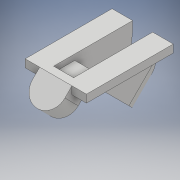
# Autodesk Inventor part: shaft_jig
Saved by Autodesk Inventor 2017 SP1 (Build 210196100, 196)
## iProperties
Part Number: shaft_jig
Material: 一般
Document SubType Name: Modeling
Designer: gisen
Density: 1 g/cm^3
Appearance: 既定
Author: gisen
Autodesk Inventor part; units mm, degrees
ref_plane "YZ Plane" through (0, 0, 0) normal (1, 0, 0) x (0, 1, 0)
ref_plane "XZ Plane" through (0, 0, 0) normal (0, 1, 0) x (-1, 0, 0)
ref_plane "XY Plane" through (0, 0, 0) normal (0, 0, 1) x (1, 0, 0)
sketch "スケッチ1" plane through (0, 0, 0) normal (0, 0, 1) x (1, 0, 0)
  line L0 (-27.5, -39) -> (27.5, -39)
  line L1 (27.5, -39) -> (27.5, 39)
  line L2 (27.5, 39) -> (-27.5, 39)
  line L3 (-27.5, 39) -> (-27.5, -39)
  line L4 (-27.5, -39) -> (27.5, 39) construction
  line L5 (27.5, -39) -> (-27.5, 39) construction
  point P0 (0, 0)
  dimension "d0" = 55
  dimension "d1" = 78
  constraints: 12 end point, 2 midpoint, 2 parallel, 1 horizontal, 1 perpendicular
  measures "d0" distance of L2.end L1.end
  measures "d1" distance of L1.end L0.end
extrude "押し出し1" add sketch "スケッチ1" along normal blind 7
sketch "スケッチ2" plane through (0, 0, 7) normal (0, 0, 1) x (1, 0, 0)
  line L0 (9, -27) -> (9, 39)
  line L1 (9, 39) -> (-9, 39)
  line L2 (-9, 39) -> (-9, -27)
  line L3 (-9, -27) -> (9, -27)
  line L4 (9, -27) -> (-9, 39) construction
  line L5 (9, 39) -> (-9, -27) construction
  point P0 (0, 0)
  point P1 (0, 6)
  dimension "d4" = 18
  dimension "d5" = 66
  dimension "d15" = 9
  constraints: 12 end point, 2 midpoint, 2 parallel, 1 perpendicular
  measures "d4" distance of L1.end L0.end
  measures "d5" distance of L0.start L0.end
  measures "d15" distance from line of L0 point (0, 0)
extrude "押し出し2" cut sketch "スケッチ2" against normal blind 7
ref_plane "作業平面1" through (-27.5, -39, 7) normal (0, 0.7071068, -0.7071068) x (1, 0, 0)
sketch "スケッチ5" plane through (-27.5, -39, 7) normal (0, 0.7071068, -0.7071068) x (1, 0, 0)
  line L0 (0, 4.9497) -> (55, 4.9497) projected
  line L1 (55, 4.9497) -> (55, 0) projected
  line L2 (0, 0) -> (55, 0) projected
  line L3 (0, 4.9497) -> (0, 0) projected
  line L4 (27.5, 9) -> (42, 9) construction
  line L5 (27.5, 9) -> (42, 9) construction
  line L6 (27.5, 9) -> (13, 9) construction
  line L7 (42, 0) -> (13, 0)
  line L8 (13, 0) -> (13, 9)
  line L9 (42, 9) -> (42, 0)
  line L10 (42, 9) -> (13, 9)
  line L11 (13, 9) -> (13, 0)
  line L12 (13, 0) -> (42, 0)
  line L13 (42, 0) -> (42, 9)
  arc A0 (42, 9) -> (13, 9) centre (27.5, 9) ccw
  point P0 (27.5, -22.6274)
  dimension "d14" = 180
  dimension "d16" = 9
  dimension "d17" = 0
  dimension "d18" = 9
  dimension "d19" = 55
  dimension "d20" = 27.5
  constraints: 20 end point, 2 horizontal, 2 parallel, 2 perpendicular, 2 point on circle, 1 centre point, 1 coincident, 1 collinear, 1 vertical
  measures "d14" angle of L6 L4
  measures "d16" distance of L5.end L7.start
  measures "d17" distance between parallel lines of L7 L2
  measures "d18" distance of L7.end L6.end
  measures "d19" distance of L0.start L0.end
  measures "d20" distance from line of L3 L4.start
extrude "押し出し4" add sketch "スケッチ5" along normal blind 17 contours L8 L10 L9 L0 | L0 L9 L2 L8 | A0 L10
sketch "スケッチ6" plane through (-14.5, -26.9792, -5.0208) normal (0, 0.7071068, 0.7071068) x (1, 0, 0)
  line L0 (5.5, -7.1005) -> (23.5, -7.1005) projected
  line L1 (29, -7.1005) -> (0, -7.1005) projected
  line L2 (29, -7.1005) -> (29, 0) projected
  line L3 (0, 0) -> (29, 0) projected
  line L4 (0, -7.1005) -> (0, 0) projected
  line L5 (0, -17) -> (0, 0) projected
  line L6 (29, -7.1005) -> (0, -7.1005)
  line L7 (0, -7.1005) -> (0, 0)
  line L8 (0, 0) -> (29, 0)
  line L9 (29, 0) -> (29, -7.1005)
  point P0 (14.5, 15.5269)
  constraints: 8 end point, 2 parallel, 1 horizontal, 1 perpendicular
extrude "押し出し5" add sketch "スケッチ6" along normal up to surface surface through (0, 0, 0) normal (0, 0, 1)
chamfer "面取り1" distance 5 angle 45 1 edges at (0, -27, 7)
sketch "スケッチ8" plane through (-9, -21.9584, 0) normal (0, 0, 1) x (1, 0, 0)
  line L0 (18, -5.0416) -> (18, 0) projected
  line L1 (0, 0) -> (18, 0) projected
  line L2 (0, 0) -> (0, -5.0416) projected
  line L3 (0, -5.0416) -> (18, -5.0416) projected
  line L4 (0, -5.0416) -> (18, -5.0416) projected
  line L5 (0, -5.0416) -> (18, -5.0416)
  line L6 (18, -5.0416) -> (18, 8.9584)
  line L7 (18, 8.9584) -> (0, 8.9584)
  line L8 (0, 8.9584) -> (0, -5.0416)
  point P0 (9, 21.9584)
  dimension "d30" = 14
  constraints: 8 end point, 2 parallel, 1 horizontal, 1 perpendicular
  measures "d30" distance of L6.end L5.end
extrude "押し出し8" add sketch "スケッチ8" along normal blind 2
ref_plane "作業平面2" through (-27.5, 1.3051, -33.3051) normal (0, 0.7071068, -0.7071068) x (-1, 0, 0)
ref_plane "作業平面3" through (7.25, -21.9584, 0) normal (0, 0.7071068, 0.7071068) x (1, 0, 0)
sketch "スケッチ9" plane through (7.25, -21.9584, 0) normal (0, 0.7071068, 0.7071068) x (1, 0, 0)
  line L0 (-21.75, 0) -> (-21.75, -12.0503) projected
  line L1 (-34.75, -12.0503) -> (-21.75, -12.0503) projected
  line L2 (-34.75, 43.1041) -> (-34.75, -12.0503) projected
  line L3 (-16.25, 43.1041) -> (-34.75, 43.1041) projected
  line L4 (-16.25, 43.1041) -> (-16.25, 6.3345) projected
  line L5 (1.75, 6.3345) -> (-16.25, 6.3345) construction
  line L6 (1.75, 6.3345) -> (1.75, 43.1041) projected
  line L7 (20.25, 43.1041) -> (1.75, 43.1041) projected
  line L8 (20.25, -12.0503) -> (20.25, 43.1041) projected
  line L9 (7.25, -12.0503) -> (20.25, -12.0503) projected
  line L10 (7.25, -12.0503) -> (7.25, 0) projected
  line L11 (-21.75, 0) -> (7.25, 0) projected
  line L12 (-7.25, 50) -> (6, 50) construction
  line L13 (-7.25, 50) -> (6, 50) construction
  line L14 (-7.25, 50) -> (-20.5, 50) construction
  line L15 (7.25, 0) -> (-21.75, 0) projected
  line L16 (6, 50) -> (6, 0)
  line L17 (-20.5, 50) -> (-20.5, 0)
  line L18 (6, 0) -> (-20.5, 0)
  line L19 (-20.5, 0) -> (6, 0)
  arc A0 (6, 50) -> (-20.5, 50) centre (-7.25, 50) ccw
  point P0 (-7.25, 15.5269)
  dimension "d40" = 50
  dimension "d41" = 26.5
  constraints: 14 end point, 3 perpendicular, 2 collinear, 2 point on circle, 2 point on line, 1 centre point, 1 coincident, 1 horizontal
  measures "d40" distance of L13.end L16.end
  measures "d41" distance between parallel lines of L17 L16
extrude "押し出し9" add sketch "スケッチ9" along normal up to surface contours L17 A0 L16 L11 surface through (0, 0, 0) normal (0, 0, 1)
sketch "スケッチ10" plane through (13.25, -21.9584, 0) normal (1, 0, 0) x (0, 0, -1)
  line L0 (-7, -17.0416) -> (0, -17.0416) projected
  line L1 (-7, -17.0416) -> (-0.636, -23.4056) projected
  line L2 (-0.636, -23.4056) -> (11.3848, -11.3848) projected
  line L3 (11.3848, -11.3848) -> (0, 0) projected
  line L4 (0, -17.0416) -> (0, 0) projected
  line L5 (0, 70.7107) -> (0, 60.9584) projected
  line L6 (0, 0) -> (0, 60.9584) projected
  line L7 (0, 0) -> (35.3553, 35.3553) projected
  line L8 (35.3553, 35.3553) -> (0, 70.7107) projected
  line L9 (0, -7.8048) -> (7, -7.8048)
  line L10 (7, -7.8048) -> (7, 11.1857)
  line L11 (7, 11.1857) -> (0, 11.1857)
  line L12 (0, 11.1857) -> (0, -7.8048)
  line L13 (0, -17.0416) -> (0, 60.9584) projected
  line L14 (0, 60.9584) -> (-7, 60.9584) projected
  line L15 (-7, -17.0416) -> (-7, 60.9584) projected
  line L16 (0, -17.0416) -> (-7, -17.0416) projected
  line L17 (0, -17.0416) -> (0, 60.9584) projected
  point P0 (0, 21.9584)
  dimension "d44" = 7
  constraints: 8 end point, 2 parallel, 2 perpendicular, 1 collinear
  measures "d44" distance of L9.start L9.end
extrude "押し出し10" add sketch "スケッチ10" against normal blind 5 contours L4 L3 L10 L9 | L7 L10 L3 | L6 L11 L10 L7
mirror "ミラー1" about plane through (0, 0, 0) normal (1, 0, 0) of "押し出し10"
sketch "スケッチ12" plane through (8.25, -21.9584, 0) normal (-1, 0, 0) x (0, 0, 1)
  line L0 (0, 0) -> (-4.2266, 4.2266)
  line L1 (-7, 7) -> (0, 0) projected
  line L2 (0, 0) -> (-7, -7) projected
  line L3 (-3.805, -3.805) -> (0, 0)
  line L4 (0, 0) -> (-5, -5)
  line L5 (-5, -5) -> (-5, 5)
  line L6 (-7, 7) -> (-7, -7) projected
  point P0 (0, 21.9584)
  dimension "d47" = 5
  constraints: 8 end point, 3 point on line, 1 collinear, 1 parallel, 1 vertical
  measures "d47" distance from line of L5 L0.start
extrude "押し出し11" add sketch "スケッチ12" along normal up to next contours L2 L5 L1 L0
ref_plane "作業平面4" through (9, -13, 2) normal (0, 0.7071068, 0.7071068) x (-1, 0, 0)
sketch "スケッチ13" plane through (0, 0, 0) normal (1, 0, 0) x (0, 1, 0)
  line L0 (39, 0) -> (39, 7) projected
  line L1 (48.7523, 0) -> (67.4906, 0) projected
  line L2 (39, 0) -> (67.4906, 0)
  line L3 (67.4906, 0) -> (39, 0)
  line L4 (39, 0) -> (35.6649, -31.8257)
  line L5 (22.7661, -44.7245) -> (67.4906, 0) projected
  line L6 (39, 0) -> (71, 0) construction
  line L7 (35.6649, -31.8257) -> (67.4906, 0)
  point P0 (0, 0)
  dimension "d54" = 32
  constraints: 10 end point, 3 collinear, 1 equal length, 1 horizontal, 1 point on line
  measures "d54" distance of L0.start L4.end
extrude "押し出し12" cut sketch "スケッチ13" along normal through all both and the other way through all
ref_plane "作業平面5" through (27.5, 39, 7) normal (0, 0.7071068, 0.7071068) x (-1, 0, 0)
sketch "スケッチ16" plane through (27.5, 39, 7) normal (0, 0.7071068, 0.7071068) x (-1, 0, 0)
  line L0 (18.5, 33.234) -> (18.5, 43.1335) projected
  line L1 (18.5, 33.234) -> (36.5, 33.234)
  line L2 (36.5, 33.234) -> (36.5, -26.766)
  line L3 (36.5, -26.766) -> (18.5, -26.766)
  line L4 (18.5, -26.766) -> (18.5, 33.234)
  point P0 (27.5, 22.6274)
  dimension "d56" = 18
  dimension "d57" = 60
  constraints: 8 end point, 2 parallel, 1 horizontal, 1 perpendicular
  measures "d56" distance of L2.end L3.end
  measures "d57" distance of L1.end L2.end
extrude "押し出し13" cut sketch "スケッチ16" against normal blind 30
sketch "スケッチ17" plane through (9, -13, 2) normal (0, 0.7071068, 0.7071068) x (-1, 0, 0)
  line L0 (0, 0) -> (18, 0) projected
  line L1 (0, 0) -> (18, 0)
  line L2 (18, 0) -> (18, -12)
  line L3 (18, -12) -> (0, -12)
  line L4 (0, -12) -> (0, 0)
  point P0 (9, -10.6066)
  dimension "d60" = 18
  dimension "d61" = 12
  constraints: 8 end point, 2 parallel, 1 horizontal, 1 perpendicular
  measures "d60" distance of L2.end L3.end
  measures "d61" distance of L1.end L2.end
sketch "スケッチ18" plane through (27.5, 17.7868, -14.2132) normal (0, 0.7071068, 0.7071068) x (1, 0, 0)
  line L0 (-18.5, 21.57) -> (-18.5, 4.9497) projected
  line L1 (-27.5, 9.0957) -> (-36.5, 9.0957)
  arc A0 (-18.5, 9.0957) -> (-36.5, 9.0957) centre (-27.5, -2.9043) ccw
  line L2 (-18.5, -43.1335) -> (-36.5, -43.1335) projected
  line L3 (-18.5, -33.234) -> (-18.5, -43.1335) projected
  line L4 (-18.5, -33.234) -> (-36.5, -33.234) projected
  line L5 (-36.5, -43.1335) -> (-36.5, -33.234) projected
  line L6 (-36.5, 9.0957) -> (-36.5, -21.234)
  line L7 (-18.5, 21.57) -> (-18.5, -20.1005) projected
  line L8 (-18.5, -31.8198) -> (-18.5, -20.1005) projected
  line L9 (-18.5, -33.234) -> (-18.5, -43.1335) projected
  line L10 (-18.5, -20.1005) -> (-18.5, -33.234)
  line L11 (-18.5, -33.234) -> (-36.5, -33.234)
  line L12 (-36.5, -33.234) -> (-36.5, -31.8198) projected
  line L13 (-36.5, -33.234) -> (-36.5, 9.0957)
  line L14 (-36.5, -20.1005) -> (-36.5, 21.57) projected
  line L15 (-18.5, 9.0957) -> (-18.5, -33.234)
  point P0 (-27.5, -22.6274)
  point P1 (-27.5, 25.0957)
  point P2 (-27.5, 12.0957)
  dimension "d62" = 13
  dimension "d63" = 3
  constraints: 12 end point, 3 point on circle, 2 collinear, 1 centre point, 1 parallel, 1 point on line, 1 vertical
  measures "d62" distance of point (-27.5, 25.096) point (-27.5, 12.096)
  measures "d63" distance of point (-27.5, 12.096) L1.start
extrude "押し出し15" add sketch "スケッチ17" against normal blind 5
extrude "押し出し16" cut sketch "スケッチ18" against normal up to surface (10.3051 mm away)
sketch "スケッチ19" plane through (9, -13, 2) normal (0, 0.7071068, 0.7071068) x (-1, 0, 0)
  line L0 (0, 0) -> (18, 0) projected
  line L1 (9, -12) -> (9, -19)
  line L2 (0, -33.234) -> (0, 16.9706) projected
  arc A0 (18, -19) -> (0, -19) centre (9, -21.2857) ccw
  arc A1 (0, -42.3297) -> (18, -42.3297) centre (9, -30.3297) ccw projected
  arc A2 (0, -42.3297) -> (18, -42.3297) centre (9, -30.3297) ccw
  line L3 (0, -54.804) -> (0, -42.3297) projected
  line L4 (0, -42.3297) -> (0, -19)
  line L5 (18, -19) -> (18, -42.3297)
  line L6 (18, 16.9706) -> (18, -33.234) projected
  point P0 (9, -10.6066)
  dimension "d71" = 12
  dimension "d72" = 7
  constraints: 6 end point, 5 point on circle, 2 centre point, 2 collinear, 1 concentric, 1 point on line, 1 vertical
  measures "d71" distance from line of L0 L1.start
  measures "d72" distance of L1.start L1.end
extrude "押し出し17" cut sketch "スケッチ19" against normal through all contours A0 L5 A1 L4 L2
sketch "スケッチ20" plane through (7.25, -21.9584, 0) normal (0, -0.7071068, -0.7071068) x (-1, 0, 0)
  arc A0 (16.25, 47.25) -> (-1.75, 47.25) centre (7.25, 35.25) ccw projected
  arc A1 (16.25, 59.7243) -> (-1.75, 59.7243) centre (7.25, 50) ccw projected
  line L0 (-1.75, 23.9203) -> (-1.75, 47.25) projected
  arc A2 (16.25, 47.25) -> (-1.75, 47.25) centre (7.25, 35.25) ccw projected
  line L1 (16.25, 47.25) -> (16.25, 23.9203) projected
  arc A3 (-1.75, 23.9203) -> (16.25, 23.9203) centre (7.25, 26.206) ccw projected
  line L2 (-1, 7.0711) -> (15.5, 7.0711) projected
  line L3 (15.5, 7.0711) -> (15.5, 9.8995) projected
  line L4 (15.5, 9.8995) -> (20.5, 9.8995) projected
  line L5 (20.5, 50) -> (20.5, 9.8995) projected
  arc A4 (20.5, 50) -> (-6, 50) centre (7.25, 50) ccw projected
  line L6 (-6, 9.8995) -> (-6, 50) projected
  line L7 (-6, 9.8995) -> (-1, 9.8995) projected
  line L8 (-1, 9.8995) -> (-1, 7.0711) projected
  line L9 (7.25, 50.25) -> (7.25, 63.25)
  circle A5 centre (7.25, 56.75) radius 4
  point P0 (7.25, 15.5269)
  dimension "d75" = 8
  constraints: 2 end point, 2 point on circle, 1 centre point, 1 coincident, 1 midpoint, 1 vertical
  measures "d75" diameter of A5
extrude "押し出し18" cut sketch "スケッチ20" against normal through all contours A5 L9 | L9 A5
thread "ねじ1" size "M8x1.25" class "6H" standard "ANSI Metric M Profile" full length
ref_plane "作業平面6" through (7.25, -12.0589, 9.8995) normal (0, -0.7071068, -0.7071068) x (-1, 0, 0)
sketch "スケッチ21" plane through (7.25, -12.0589, 9.8995) normal (0, -0.7071068, -0.7071068) x (-1, 0, 0)
  line L0 (20.5, 50) -> (20.5, 9.8995) projected
  line L1 (20.5, 43.1041) -> (20.5, 0) projected
  line L2 (20.5, 14) -> (20.5, 34)
  line L3 (20.5, 14) -> (29.5, 14)
  line L4 (20.5, 14) -> (29.5, 14) construction
  line L5 (29.5, 14) -> (20.5, 34)
  point P0 (7.25, 15.5269)
  dimension "d83" = 20
  dimension "d84" = 9
  dimension "d85" = 0
  constraints: 8 end point, 2 point on line, 1 collinear, 1 horizontal, 1 perpendicular
  measures "d83" distance of L2.start L2.end
  measures "d84" distance of L2.start L3.end
  measures "d85" distance between parallel lines of L4 L3
extrude "押し出し19" add sketch "スケッチ21" against normal blind 3
sketch "スケッチ22" plane through (-13.25, -28.9584, -7) normal (-1, 0, 0) x (0, 0, 1)
  line L0 (7, 67.9584) -> (-3.8939, 66.8168) projected
  line L1 (-28.3553, 42.3553) -> (-3.8939, 66.8168) projected
  line L2 (-28.3553, 42.3553) -> (0, 14) projected
  line L3 (0, 0) -> (0, 14) projected
  line L4 (7, 7) -> (0, 0) projected
  line L5 (7, 67.9584) -> (7, 31.0416) projected
  line L6 (-28.3553, 42.3553) -> (0, 14) projected
  line L7 (-2.8995, 16.8995) -> (7, 26.799)
  line L8 (9, 15.9584) -> (-4.435, 29.3934) projected
  line L9 (-2.8995, 16.8995) -> (11.1005, 16.8995) construction
  line L10 (7, 67.9584) -> (7, -10.0416) projected
  line L11 (-5.0208, 43.0624) -> (7, 31.0416) projected
  line L12 (7, 26.799) -> (7, 7) projected
  line L13 (7, 26.799) -> (-7.1421, 40.9411) projected
  line L14 (-7.1421, 40.9411) -> (-5.0208, 43.0624) projected
  point P0 (7, 28.9584)
  dimension "d81" = 14
  dimension "d82" = 45
  constraints: 4 end point, 2 point on line, 1 coincident, 1 equal length, 1 horizontal, 1 perpendicular
  measures "d81" distance of L7.start L7.end
  measures "d82" angle of L9 L7
mirror "ミラー2" about plane through (0, 0, 0) normal (1, 0, 0) of "押し出し19"
equation "\"d15\" = 0.5 * d4"
equation "\"d20\" = 0.5 * d19"
